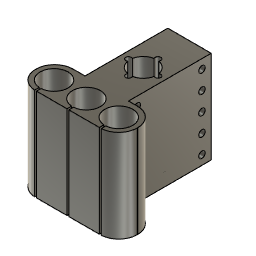
X-Carriage (Autodesk Fusion 360 design; units mm, degrees)
Autodesk Fusion 360 part; units mm, degrees
sketch "Skizze1" plane through (0, 0, 0) normal (0, 0, 1) x (1, 0, 0)
  circle A0 centre (0, 0) radius 7.55
  line L0 (27.5, -10) -> (-11, -10)
  line L1 (-11, -10) -> (-11, 55)
  line L2 (-11, 55) -> (27.5, 55)
  line L3 (27.5, 55) -> (27.5, -10)
  line L4 (0, 0) -> (0, -10)
  line L5 (0, -10) -> (-0.5, -10)
  line L6 (-0.5, -10) -> (0.5, -10)
  line L7 (0.5, -10) -> (0.5, -5)
  line L8 (0.5, -5) -> (-0.5, -5)
  line L9 (-0.5, -5) -> (-0.5, -10)
  circle A1 centre (0.75, 30) radius 6.5
  circle A2 centre (0.75, 30) radius 8
  line L10 (0.75, 30) -> (0.75, 38)
  line L11 (0.75, 30) -> (8.75, 30)
  line L12 (0.75, 30) -> (0.75, 22)
  line L13 (0.75, 30) -> (-7.25, 30)
  circle A3 centre (0.75, 38) radius 1.5
  circle A4 centre (8.75, 30) radius 1.5
  circle A5 centre (0.75, 22) radius 1.5
  circle A6 centre (-7.25, 30) radius 1.5
  circle A7 centre (0.75, 30) radius 11.4
  circle A8 centre (17.5, 0) radius 7.55
  line L14 (17, -10) -> (18, -10)
  line L15 (18, -10) -> (18, -5)
  line L16 (18, -5) -> (17, -5)
  line L17 (17, -5) -> (17, -10)
  line L18 (27.5, 55) -> (12.5, 55)
  line L19 (12.5, 55) -> (12.5, 10.25)
  line L20 (12.5, 10.25) -> (27.5, 10.25)
  line L21 (27.5, 10.25) -> (27.5, 55)
  line L22 (27.5, 10.25) -> (17.5, 0.25)
  line L23 (27.5, 10.25) -> (56.3877, 10.25) construction
  line L24 (17.5, 0) -> (17.5, 0.25)
  arc A9 (27.5, -2.25) -> (15, 10.25) centre (15, -2.25) ccw
  circle A10 centre (-17.5, 0) radius 7.55
  line L25 (-11, -10) -> (-27.5, -10)
  line L26 (-27.5, -10) -> (-27.5, 10.25)
  line L27 (-27.5, 10.25) -> (-11, 10.25)
  line L28 (-11, 10.25) -> (-11, -10)
  line L29 (-18, -5) -> (-17, -5)
  line L30 (-17, -5) -> (-17, -10)
  line L31 (-17, -10) -> (-18, -10)
  line L32 (-18, -10) -> (-18, -5)
  dimension "d1" = 15.1
  dimension "d5" = 10
  dimension "d6" = 11
  dimension "d7" = 65
  dimension "d15" = 13
  dimension "d17" = 16
  dimension "d18" = 3
  dimension "d19" = 22.8
  dimension "d38" = 5
  dimension "d45" = 15.1
  dimension "d47" = 5
  dimension "d48" = 0.5
  dimension "d49" = 12.5
  dimension "d50" = 10.25
  dimension "d58" = 135
  dimension "d61" = 17.5
  dimension "d62" = 10
  dimension "d63" = 11.75
  dimension "d64" = 30
  dimension "d69" = 17.5
  dimension "d70" = 10
  dimension "d71" = 10
  dimension "d72" = 1
  dimension "d73" = 17.5
  constraint coincident A0.centre L4.start
  constraint horizontal L0
  constraint vertical L1
  constraint horizontal L2
  constraint vertical L3
  constraint coincident L0 L4.end
  constraint perpendicular L0 L4
  constraint coincident L0 L5.end
  constraint horizontal L6
  constraint vertical L7
  constraint horizontal L8
  constraint vertical L9
  constraint concentric A1 A2
  constraint coincident A1.centre A2.centre
  constraint vertical L10
  constraint perpendicular L10 L11
  constraint coincident A2 L12.end
  constraint parallel L10 L12
  constraint coincident A2 L13.end
  constraint perpendicular L12 L13
  constraint coincident A2 L10.end
  constraint coincident A2 L11.end
  constraint coincident L10.end A3.centre
  constraint coincident L11.end A4.centre
  constraint coincident L12.end A5.centre
  constraint coincident L13.end A6.centre
  constraint equal A3 A4
  constraint equal A3 A6
  constraint equal A3 A5
  constraint concentric A1 A7
  constraint horizontal L14
  constraint vertical L15
  constraint horizontal L16
  constraint vertical L17
  constraint coincident L0 L14.start
  constraint equal L8 L16
  constraint horizontal L18
  constraint vertical L19
  constraint horizontal L20
  constraint vertical L21
  constraint horizontal L23
  constraint coincident A8.centre L24.start
  constraint vertical L24
  constraint coincident L20 A9.end
  constraint coincident L3 A9.start
  constraint equal A0 A10
  constraint horizontal L25
  constraint vertical L26
  constraint horizontal L27
  constraint vertical L28
  constraint collinear L20 L27
  constraint horizontal L29
  constraint vertical L30
  constraint horizontal L31
  constraint vertical L32
  constraint equal L9 L30
  constraint collinear L0 L31
  measures "d1" diameter of A0
  measures "d5" distance of A0.centre L0
  measures "d6" distance of A0.centre L1
  measures "d7" distance of L0.start L2.end
  measures "d15" diameter of A1
  measures "d17" diameter of A2
  measures "d18" diameter of A3
  measures "d19" diameter of A7
  measures "d38" vertical distance of A0.centre L7.end
  measures "d45" diameter of A8
  measures "d47" distance of A8.centre L16
  measures "d48" distance of A8.centre L17
  measures "d49" distance of A0.centre L19
  measures "d50" distance of A8.centre L20
  measures "d58" angle of L22 L23
  measures "d61" distance of A0.centre A8.centre
  measures "d62" distance of L3 A8.centre
  measures "d63" distance of L1 A1.centre
  measures "d64" vertical distance of A0.centre A1.centre
  measures "d69" distance of A0.centre A10.centre
  measures "d70" distance of A10.centre L25
  measures "d71" distance of A10.centre L26
  measures "d72" distance of L29.start L29.end
  measures "d73" distance of L7 L30
extrude "Extrusion1" add sketch "Skizze1" along normal blind 50 contours A0 L0 L1 L2 L7 L9 A8 L17 L19 L20 L22 A9 A10 L28 | L1 A10 L25 L28 L30 | L0 L3 A8 L15 L22 A9 | L1 A10 L25 L26 L27 L28 L32 | L3 L22 A9 | L20 L22 A9 | A1 A2 A4 A5 | A1 A2 A3 A4 | A1 A2 A3 A6 | A1 A2 A5 A6 | A7
extrude "Extrusion3" cut sketch "Skizze1" along normal blind 7 contours A1 L10 L11 | A1 A2 A4 A5 | A1 L11 L12 | A1 A2 A3 A4 | A1 L10 L13 | A1 A2 A3 A6 | A1 A2 A5 A6 | A1 L12 L13 | A7
sketch "Skizze3" plane through (-11, 0, 0) normal (-1, 0, 0) x (0, -1, 0)
  line L0 (-55, 0) -> (-10.25, 0)
  line L1 (-10.25, 50) -> (-55, 50)
  line L2 (-55, 50) -> (-55, 0)
  line L3 (-50, 45) -> (-15, 45)
  line L4 (-15, 45) -> (-15, 5)
  line L5 (-15, 5) -> (-50, 5)
  line L6 (-50, 5) -> (-50, 45)
  circle A0 centre (-50, 45) radius 1.75
  circle A1 centre (-15, 45) radius 1.75
  circle A2 centre (-15, 5) radius 1.75
  circle A3 centre (-50, 5) radius 1.75
  circle A4 centre (-50, 25) radius 1.75
  circle A5 centre (-15, 25) radius 1.75
  line L7 (-50, 45) -> (-50, 35)
  line L8 (-50, 5) -> (-50, 15)
  line L9 (-15, 45) -> (-15, 35)
  line L10 (-15, 5) -> (-15, 15)
  circle A6 centre (-50, 35) radius 1.75
  circle A7 centre (-15, 35) radius 1.75
  circle A8 centre (-15, 15) radius 1.75
  circle A9 centre (-50, 15) radius 1.75
  line L11 (-15, 45) -> (-15, 5)
  line L12 (-10.25, 0) -> (-10.25, 50)
  dimension "d23" = 5
  dimension "d24" = 5
  dimension "d25" = 5
  dimension "d28" = 3.5
  dimension "d31" = 10
  dimension "d32" = 10
  dimension "d33" = 10
  dimension "d34" = 10
  dimension "d67" = 35
  constraint horizontal L3
  constraint vertical L4
  constraint horizontal L5
  constraint vertical L6
  constraint coincident L3.start L6.end
  constraint coincident L3.end L4.start
  constraint coincident L4.end L5.start
  constraint coincident L5.end L6.start
  constraint equal A0 A3
  constraint equal A0 A1
  constraint equal A0 A2
  constraint midpoint L6 A4.centre
  constraint midpoint L4 A5.centre
  constraint equal A0 A4
  constraint equal A0 A5
  constraint perpendicular L3 L7
  constraint perpendicular L5 L8
  constraint perpendicular L3 L9
  constraint perpendicular L5 L10
  constraint coincident L7.end A6.centre
  constraint coincident L9.end A7.centre
  constraint coincident L10.end A8.centre
  constraint coincident L8.end A9.centre
  constraint equal A0 A6
  constraint equal A0 A9
  constraint equal A0 A7
  constraint equal A0 A8
  constraint vertical L11
  measures "d23" distance of L1 L3
  measures "d24" distance of L0 L5
  measures "d25" distance of L2 L6
  measures "d28" diameter of A0
  measures "d31" distance of L3.start L7.end
  measures "d32" distance of L5.end L8.end
  measures "d33" distance of L3.end L9.end
  measures "d34" distance of L4.end L10.end
  measures "d67" distance of L3.start L3.end
extrude "Extrusion4" cut sketch "Skizze3" against normal blind 45 contours L3 L6 A0 L7 | L3 L6 A0 L7 | L3 L4 A1 L9 L11 | L3 L4 A1 L9 L11 | L6 L7 A6 | L6 L7 A6 | L4 L9 A7 L11 | L4 L9 A7 L11 | L6 A4 | L6 A4 | L4 A5 L11 | L4 A5 L11 | L6 L8 A9 | L6 L8 A9 | L4 L10 A8 L11 | L4 L10 A8 L11 | L5 L6 A3 L8 | L5 L6 A3 L8 | L4 L5 A2 L10 L11 | L4 L5 A2 L10 L11
sketch "Skizze6" plane through (0, 0, 50) normal (0, 0, 1) x (-1, 0, 0)
  line L0 (-12.5, -10.25) -> (-12.5, -55)
  line L1 (-12.5, -55) -> (11, -55)
  line L2 (17, 10) -> (0.5, 10)
  line L3 (0.5, 10) -> (0.5, 7.5334)
  arc A0 (-0.5, 7.5334) -> (0.5, 7.5334) centre (0, 0) ccw
  line L4 (-0.5, 7.5334) -> (-0.5, 10)
  line L5 (-0.5, 10) -> (-17, 10)
  line L6 (-17, 10) -> (-17, 7.5334)
  arc A1 (-18, 7.5334) -> (-17, 7.5334) centre (-17.5, 0) ccw
  line L7 (-18, 7.5334) -> (-18, 10)
  line L8 (-18, 10) -> (-27.5, 10)
  line L9 (-27.5, 10) -> (-27.5, -10.25)
  line L10 (-27.5, -10.25) -> (-12.5, -10.25)
  circle A2 centre (-0.75, -30) radius 7.25
  circle A3 centre (-0.75, -38) radius 1.5
  circle A4 centre (-8.75, -30) radius 1.5
  circle A5 centre (7.25, -30) radius 1.5
  circle A6 centre (-0.75, -22) radius 1.5
  arc A7 (-7.25, -29.9997) -> (-0.75, -36.5) centre (-0.75, -30) ccw
  arc A8 (-0.75, -23.5) -> (-7.25, -29.9997) centre (-0.75, -30) ccw
  arc A9 (-0.75, -36.5) -> (5.75, -30) centre (-0.75, -30) ccw
  arc A10 (5.75, -30) -> (-0.75, -23.5) centre (-0.75, -30) ccw
  line L11 (27.5, -10.25) -> (27.5, 10)
  line L12 (11, -55) -> (11, -10.25)
  line L13 (11, -10.25) -> (27.5, -10.25)
  line L14 (27.5, 10) -> (18, 10)
  line L15 (18, 10) -> (18, 7.5334)
  arc A11 (17, 7.5334) -> (18, 7.5334) centre (17.5, 0) ccw
  line L16 (17, 7.5334) -> (17, 10)
  dimension "d51" = 14.5
  constraint coincident A2.centre A7.centre
  measures "d51" diameter of A2
extrude "Extrusion7" cut sketch "Skizze6" against normal blind 30 contours A2 A5 A6 A10 | A2 A3 A5 A9 | A7 A8 A9 A10 | A2 A3 | A2 A4 A6 A8 | A2 A3 A4 A7 | A2 A4 picked at (-0.75, -36.9922) picked at (-7.7422, -30)
chamfer "Fase2" distance 0.75 angle 45 4 edges at (-4.3765, 24.8735, 20) (-4.3765, 35.1265, 20) (5.8765, 35.1265, 20) (5.8765, 24.8735, 20)
fillet "Abrundung1" radius 10 4 edges at (27.5, 10.25, 25) (27.5, -10, 25) (-27.5, -10, 25) (-27.5, 10.25, 25)
equation "d50 = ( 20.5 / 2 ) * 1 mm"
equation "d63 = ( 23.5 / 2 ) * 1 mm"
